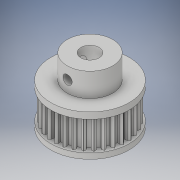
# Autodesk Inventor part: SmallBelt_Pulley
Saved by Autodesk Inventor 2019.4 (Build 234330000, 330)
## iProperties
Created: 2021-02-02
Part Number: SmallBelt_Pulley
Material: Generic
Document SubType Name: Modeling
Designer: Jorian Brusind
Density: 1 g/cm^3
Appearance: Default
Author: Jorian Brusind
Autodesk Inventor part; units mm, degrees
ref_plane "YZ Plane" through (0, 0, 0) normal (1, 0, 0) x (0, 1, 0)
ref_plane "XZ Plane" through (0, 0, 0) normal (0, 1, 0) x (-1, 0, 0)
ref_plane "XY Plane" through (0, 0, 0) normal (0, 0, 1) x (1, 0, 0)
sketch "Sketch1" plane through (0, 0, 0) normal (0, 1, 0) x (-1, 0, 0)
  circle A0 centre (0, 0) radius 10.75
  dimension "d0" = 21.5
  constraints: 1 centre point, 1 coincident
  measures "d0" diameter of A0
extrude "Extrusion1" add sketch "Sketch1" along normal blind 11.25
sketch "Sketch2" plane through (0, 11.25, 0) normal (0, 1, 0) x (1, 0, 0)
  circle A0 centre (0, 0) radius 6.25
  dimension "d3" = 12.5
  constraints: 1 centre point, 1 coincident
  measures "d3" diameter of A0
extrude "Extrusion2" add sketch "Sketch2" along normal blind 6.5
sketch "Sketch3" plane through (0, 0, 0) normal (1, 0, 0) x (0, 1, 0)
  line L0 (0, 10.75) -> (0, -10.75) projected
  line L1 (0, -10.75) -> (1.5, -10.75)
  line L2 (1.5, -10.75) -> (1.5, -9)
  line L3 (0, -10.75) -> (11.25, -10.75) projected
  line L4 (1.5, -9) -> (9.5, -9)
  line L5 (9.5, -9) -> (9.5, -10.75)
  line L6 (1.5, -10.75) -> (9.5, -10.75)
  line L7 (17.75, -6.25) -> (17.75, 6.25) projected
  line L8 (17.75, 0) -> (0, 0)
  dimension "d6" = 1.5
  dimension "d7" = 1.75
  dimension "d8" = 8
  constraints: 12 end point, 5 perpendicular, 1 horizontal, 1 midpoint, 1 point on line
  measures "d6" distance of L0.end L1.end
  measures "d7" distance of L1.end L2.end
  measures "d8" distance of L2.end L4.end
revolve "Revolution1" cut sketch "Sketch3" angle 360 about axis through (0, 17.75, 0) along (0, -1, 0)
sketch "Sketch4" plane through (0, 0, 0) normal (1, 0, 0) x (0, 1, 0)
  line L0 (1.5, 10.75) -> (1.5, -10.75) projected
  line L1 (1.5, -10.75) -> (1.5, -10.25)
  line L2 (1.5, -10.25) -> (9.5, -10.25)
  line L3 (9.5, -10.25) -> (9.5, -8.75)
  line L4 (9.5, -8.75) -> (1.5, -8.75)
  line L5 (1.5, -8.75) -> (1.5, -10.25)
  line L6 (0, 0) -> (17.75, 0)
  line L7 (17.75, -6.25) -> (17.75, 6.25) projected
  dimension "d10" = 0.5
  dimension "d11" = 8
  dimension "d12" = 1.5
  constraints: 12 end point, 2 parallel, 1 horizontal, 1 midpoint, 1 perpendicular, 1 point on line
  measures "d10" distance of L0.end L1.end
  measures "d11" distance of L4.end L3.end
  measures "d12" distance of L3.end L2.end
revolve "Revolution2" add sketch "Sketch4" angle 5.805 about axis through (0, 0, 0) along (0, -1, 0)
chamfer "Chamfer1" distance 0.5 angle 45 2 edges at (1.0367, 5.5, -10.1974) (0, 5.5, -10.25)
pattern_circular "Circular Pattern1" count 31 over 360 about axis through (0, 5.5, 0) along (0, 1, 0) of "Revolution2", "Chamfer1"
sketch "Sketch5" plane through (0, 17.75, 0) normal (0, 1, 0) x (1, 0, 0)
  circle A0 centre (0, 0) radius 2.5
  dimension "d20" = 5
  constraints: 1 centre point, 1 coincident
  measures "d20" diameter of A0
extrude "Extrusion3" cut sketch "Sketch5" against normal up to next
sketch "Sketch6" plane through (0, 0, 0) normal (1, 0, 0) x (0, 1, 0)
  line L0 (17.75, 2.5) -> (17.75, -2.5) projected
  line L1 (17.75, 0) -> (14.45, 0)
  circle A0 centre (14.45, 0) radius 1.25
  point P0 (0, 0)
  dimension "d23" = 3.3
  dimension "d24" = 2.5
  constraints: 2 end point, 1 centre point, 1 coincident, 1 horizontal, 1 midpoint
  measures "d23" distance of L1.start L1.end
  measures "d24" diameter of A0
extrude "Extrusion4" cut sketch "Sketch6" against normal up to next
pattern_circular "Circular Pattern2" count 2 over 90 about axis through (0, 11.25, 0) along (0, 1, 0) of "Extrusion4"
body "Solid1"
